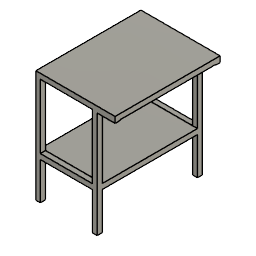
table (Autodesk Fusion 360 design; units mm, degrees)
part number: 2026-08-19-13-15-43-952
Autodesk Fusion 360 part; units mm, degrees
sketch "FrontProfile" plane through (0, 0, 0) normal (1, 0, 0) x (0, 1, 0)
  line L0 (0, 0) -> (-450, 0)
  line L1 (0, 0) -> (450, 0)
  line L2 (-450, 0) -> (-500, 0)
  line L3 (450, 0) -> (500, 0)
  line L4 (-500, 0) -> (-500, 1067)
  line L5 (500, 0) -> (500, 1066.8)
  line L6 (453.6078, 0) -> (453.6078, 1016)
  line L7 (-450, 0) -> (-450, 1016)
  line L8 (-450, 355.6) -> (453.6078, 355.6)
  line L9 (-450, 405.6) -> (453.6078, 405.6)
  line L10 (-450, 1016) -> (453.6078, 1016)
  line L11 (-500, 1067) -> (500, 1066.8)
  constraint coincident L0.start L1.start
  constraint horizontal L0
  constraint parallel L0 L1
  constraint parallel L0 L2
  constraint horizontal L3
  constraint perpendicular L2 L4
  constraint perpendicular L3 L5
  constraint coincident L3 L6.start
  constraint perpendicular L3 L6
  constraint perpendicular L0 L7
  constraint coincident L7 L8.start
  constraint coincident L6 L8.end
  constraint perpendicular L6 L8
  constraint coincident L7 L9.start
  constraint coincident L6 L9.end
  constraint perpendicular L6 L9
sketch "Sketch3" plane through (0, 0, 0) normal (0, 1, 0) x (1, 0, 0)
  line L0 (0, 0) -> (-165.5064, 0)
  line L1 (-165.5064, 0) -> (-165.5064, -1016.5)
  line L2 (0, -1100) -> (-762, -1100)
  line L3 (-165.5064, 0) -> (-216.3064, 0)
  line L4 (-216.3064, 0) -> (-216.3064, -1000)
  line L5 (-762, -1100) -> (-762, 0)
  line L6 (-762, 0) -> (-711, 0)
  line L7 (-711, 0) -> (-711, -1018.0594)
  line L8 (-711, -1018.0594) -> (-165.5064, -1016.5)
  line L9 (-216.3064, -1000) -> (-216.2588, -1016.6451)
  line L10 (0, -1100) -> (0, 0)
  line L11 (-711, -356) -> (-216.3064, -356)
  line L12 (-711, 0) -> (-216.3064, 0)
  line L13 (-216.3064, -406) -> (-711, -406)
  constraint coincident L0.start L10.end
  constraint horizontal L0
  constraint perpendicular L0 L1
  constraint perpendicular L1 L2
  constraint perpendicular L1 L3
  constraint perpendicular L2 L4
  constraint perpendicular L2 L5
  constraint perpendicular L4 L6
  constraint perpendicular L6 L7
  constraint coincident L8 L9.end
  constraint perpendicular L8 L9
  constraint perpendicular L0 L10
  constraint coincident L7 L11.start
  constraint coincident L4 L11.end
  constraint perpendicular L4 L11
  constraint perpendicular L4 L12
  constraint coincident L4 L13.start
  constraint coincident L7 L13.end
  constraint perpendicular L7 L13
sketch "Sketch4" plane through (0, 0, 0) normal (0, 0, 1) x (1, 0, 0)
  line L0 (0, 0) -> (-762, 0)
  line L1 (0, 0) -> (0, 473.2266)
  line L2 (0, 0) -> (0, 422)
  line L3 (0, 0) -> (0, -422)
  line L4 (0, -422) -> (-750.4023, -422)
  line L5 (-750.4023, -422) -> (-762, 0)
  line L6 (0, 473.2266) -> (-750.4023, 473.2266)
  line L7 (-750.4023, 473.2266) -> (-762, 0)
  line L8 (-762, 0) -> (-762, 473.2266)
  line L9 (-762, 473.2266) -> (-750.4023, 473.2266)
  line L10 (-762, 0) -> (-762, -420)
  line L11 (-762, -420) -> (-762, -422)
  line L12 (-762, -422) -> (-697, -422)
  constraint coincident L0.start L1.start
  constraint horizontal L0
  constraint perpendicular L0 L1
  constraint perpendicular L0 L2
  constraint perpendicular L0 L3
  constraint perpendicular L3 L4
  constraint perpendicular L1 L6
  constraint perpendicular L6 L8
  constraint parallel L6 L9
  constraint perpendicular L0 L10
  constraint perpendicular L4 L11
  constraint coincident L4 L12.end
  constraint perpendicular L11 L12
extrude "Extrude1" add sketch "FrontProfile" against normal blind 754 contours L2 L3 L4 L5 L6 L7 L10 L11
extrude "Extrude2" add sketch "FrontProfile" against normal blind 754 contours L6 L7 L8 L9
sketch "Sketch5" plane through (0, 0, 0) normal (0, 1, 0) x (1, 0, 0)
  line L0 (-170, -1010) -> (0, -1010)
  line L1 (-170, -1010) -> (-170, 0)
  constraint horizontal L0
  constraint perpendicular L0 L1
sketch "Sketch6" plane through (0, 500, 0) normal (0, 1, 0) x (-1, 0, 0)
  line L0 (0, 1066.8) -> (0, 0)
  line L1 (0, 0) -> (754, 0)
  line L2 (754, 0) -> (754, 1066.8)
  line L3 (754, 1066.8) -> (0, 1066.8)
  line L4 (0, 1010) -> (170, 1010)
  line L5 (170, 1010) -> (170, 0)
  line L6 (170, 0) -> (0, 0)
  line L7 (0, 0) -> (0, 1010)
  constraint coincident L0 L4.start
  constraint perpendicular L0 L4
  constraint coincident L1 L5.end
  constraint perpendicular L1 L5
  constraint coincident L0.end L1.start
extrude "Extrude3" cut sketch "Sketch6" against normal blind 1000 contours L0 L1 L4 L5 L6 L7
extrude "Extrude4" cut sketch "Sketch3" along normal blind 600 contours L4 L7 L8 L9 L13
extrude "Extrude5" cut sketch "Sketch3" against normal blind 700 contours L4 L7 L8 L9 L13
extrude "Extrude6" cut sketch "Sketch3" against normal blind 650 contours L4 L7 L11 L12
extrude "Extrude7" cut sketch "Sketch3" along normal blind 600 contours L4 L7 L11 L12
